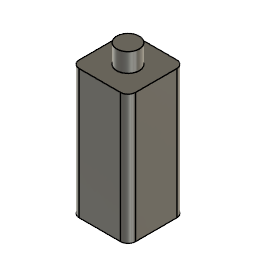
ScreenMount (Autodesk Fusion 360 design; units mm, degrees)
Autodesk Fusion 360 part; units mm, degrees
sketch "Sketch1" plane through (0, 0, 0) normal (0, 0, 1) x (1, 0, 0)
  line L0 (0, 0) -> (0, 6)
  line L1 (0, 6) -> (6, 6)
  line L2 (6, 6) -> (6, 0)
  line L3 (6, 0) -> (0, 0)
  dimension "d1" = 6
  dimension "d2" = 6
  constraint coincident L0.start L3.end
  constraint vertical L0
  constraint perpendicular L0 L1
  constraint perpendicular L1 L2
  constraint perpendicular L0 L3
  measures "d1" distance of L0.start L0.end
  measures "d2" distance of L0.end L1.end
extrude "Extrude1" add sketch "Sketch1" along normal blind 13.75
sketch "Sketch2" plane through (0, 0, 13.75) normal (0, 0, 1) x (-1, 0, 0)
  line L0 (-6, 0) -> (-6, -6)
  line L1 (-6, -6) -> (0, -6)
  line L2 (0, -6) -> (0, 0)
  line L3 (0, 0) -> (-6, 0)
  circle A0 centre (-3, -3) radius 1.2
  dimension "d6" = 2.4
  measures "d6" diameter of A0
extrude "Extrude2" add sketch "Sketch2" along normal blind 2 contours A0
sketch "Sketch3" plane through (0, 0, 0) normal (0, 0, -1) x (1, 0, 0)
  line L0 (6, -6) -> (6, 0)
  line L1 (6, 0) -> (0, 0)
  line L2 (0, 0) -> (0, -6)
  line L3 (0, -6) -> (6, -6)
  circle A0 centre (3, -3) radius 1.4
  dimension "d9" = 2.8
  measures "d9" diameter of A0
extrude "Extrude3" cut sketch "Sketch3" against normal blind 12 contours A0
fillet "Fillet1" radius 0.8 4 edges at (6, 0, 6.875) (6, 6, 6.875) (0, 6, 6.875) (0, 0, 6.875)
